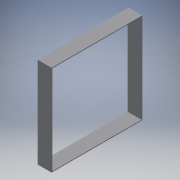
# Autodesk Inventor part: Walls
Saved by Autodesk Inventor 2019 (Build 230136000, 136)
## iProperties
Created: 2018-09-21
Part Number: Walls
Material: Generic
Document SubType Name: Modeling
Designer: user
Density: 1 g/cm^3
Appearance: Default
Author: user
Autodesk Inventor part; units mm, degrees
ref_plane "YZ Plane" through (0, 0, 0) normal (1, 0, 0) x (0, 1, 0)
ref_plane "XZ Plane" through (0, 0, 0) normal (0, 1, 0) x (-1, 0, 0)
ref_plane "XY Plane" through (0, 0, 0) normal (0, 0, 1) x (1, 0, 0)
sketch "Sketch1" plane through (0, 0, 0) normal (0, 0, 1) x (1, 0, 0)
  line L0 (0, 0) -> (-381, 0)
  line L1 (-381, 0) -> (-381, 2438.4)
  line L2 (-381, 2438.4) -> (0, 2438.4)
  line L3 (0, 2438.4) -> (0, 0)
  dimension "d0" = 2438.4
  dimension "d1" = 381
  constraints: 8 end point, 2 parallel, 1 horizontal, 1 perpendicular
  measures "d0" distance of L0.end L1.end
  measures "d1" distance between parallel lines of L3 L1
extrude "Extrusion1" add sketch "Sketch1" along normal blind 19.05
sketch "Sketch2" plane through (-381, 2438.4, 0) normal (0, 1, 0) x (1, 0, 0)
  line L0 (381, 0) -> (381, 2438.4) projected
  line L1 (381, -19.05) -> (0, -19.05) projected
  line L2 (381, -19.05) -> (0, -19.05)
  line L3 (0, -19.05) -> (0, 2438.4)
  line L4 (0, 2438.4) -> (381, 2438.4)
  line L5 (381, 2438.4) -> (381, -19.05)
  constraints: 8 end point, 2 parallel, 1 horizontal, 1 perpendicular
extrude "Extrusion2" add sketch "Sketch2" along normal blind 19.05
sketch "Sketch3" plane through (0, 2438.4, -2438.4) normal (0, 0, -1) x (-1, 0, 0)
  line L0 (0, 0) -> (0, -2438.4) projected
  line L1 (0, 19.05) -> (381, 19.05) projected
  line L2 (0, 19.05) -> (381, 19.05)
  line L3 (381, 19.05) -> (381, -2438.4)
  line L4 (381, -2438.4) -> (0, -2438.4)
  line L5 (0, -2438.4) -> (0, 19.05)
  constraints: 8 end point, 2 parallel, 1 horizontal, 1 perpendicular
extrude "Extrusion3" add sketch "Sketch3" along normal blind 19.05
sketch "Sketch4" plane through (-381, 0, -2438.4) normal (0, -1, 0) x (1, 0, 0)
  line L0 (0, 0) -> (381, 0) projected
  line L1 (0, 0) -> (0, -19.05) projected
  line L2 (381, -19.05) -> (0, -19.05) projected
  line L3 (381, 0) -> (381, -19.05) projected
  line L4 (0, 2457.45) -> (381, 2457.45) projected
  line L5 (381, 0) -> (381, -19.05) projected
  line L6 (381, -19.05) -> (0, -19.05)
  line L7 (0, -19.05) -> (0, 2457.45)
  line L8 (0, 2457.45) -> (381, 2457.45)
  line L9 (381, 2457.45) -> (381, -19.05)
  point P0 (381, 2438.4)
  constraints: 8 end point, 2 parallel, 1 horizontal, 1 perpendicular
extrude "Extrusion4" add sketch "Sketch4" along normal blind 19.05 contours L7 L4 L9 L0
body "Solid1"
